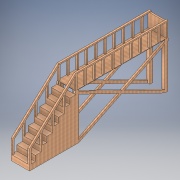
# Autodesk Inventor part: driver stand
Saved by Autodesk Inventor 2019 (Build 230136000, 136)
## iProperties
Created: 2020-04-29
Part Number: driver stand
Material: Wood (Birch)
Document SubType Name: Modeling
Designer: infinity
Density: 0.55 g/cm^3
Appearance: Birch - Natural Polished
Author: infinity
Autodesk Inventor part; units mm, degrees
ref_plane "YZ Plane" through (0, 0, 0) normal (1, 0, 0) x (0, 1, 0)
ref_plane "XZ Plane" through (0, 0, 0) normal (0, 1, 0) x (-1, 0, 0)
sketch "Sketch1" plane through (0, 0, 0) normal (0, 1, 0) x (-1, 0, 0)
  line L0 (0, 0) -> (1219.2, 0)
  line L1 (1219.2, 0) -> (1219.2, -6096)
  line L2 (1219.2, -6096) -> (0, -6096)
  line L3 (0, -6096) -> (0, 0)
  dimension "d0" = 6096
  dimension "d1" = 1219.2
  constraints: 8 end point, 2 parallel, 1 horizontal, 1 perpendicular
  measures "d0" distance of L0.end L1.end
  measures "d1" distance of L0.start L0.end
extrude "Extrusion1" add sketch "Sketch1" along normal blind 25.4
sketch "Sketch2" plane through (0, 0, 0) normal (0, -1, 0) x (1, 0, 0)
  line L0 (-1219.2, 0) -> (0, 0) projected
  line L1 (0, 0) -> (-203.2, 0)
  line L2 (-203.2, 0) -> (-203.2, -203.2)
  line L3 (-203.2, -203.2) -> (0, -203.2)
  line L4 (0, -203.2) -> (0, 0)
  line L5 (0, 0) -> (0, -6096) projected
  line L6 (0, -6096) -> (-203.2, -6096)
  line L7 (-203.2, -6096) -> (-203.2, -5892.8)
  line L8 (-203.2, -5892.8) -> (0, -5892.8)
  line L9 (0, -5892.8) -> (0, -6096)
  line L10 (0, -6096) -> (-1219.2, -6096) projected
  line L11 (-1219.2, -6096) -> (-994.7173, -6096)
  line L12 (-994.7173, -6096) -> (-994.7173, -5892.8)
  line L13 (-994.7173, -5892.8) -> (-1219.2, -5892.8)
  line L14 (-1219.2, -5892.8) -> (-1219.2, -6096)
  line L15 (-1219.2, 0) -> (-994.7173, 0)
  line L16 (-994.7173, 0) -> (-994.7173, -203.2)
  line L17 (-994.7173, -203.2) -> (-1219.2, -203.2)
  line L18 (-1219.2, -203.2) -> (-1219.2, 0)
  line L19 (-203.2, -203.2) -> (-994.7173, -203.2) construction
  line L20 (-994.7173, -203.2) -> (-994.7173, -5892.8) construction
  line L21 (-994.7173, -5892.8) -> (-203.2, -5892.8) construction
  line L22 (-203.2, -5892.8) -> (-203.2, -203.2) construction
  dimension "d4" = 203.2
  dimension "d5" = 203.2
  dimension "d6" = 203.2
  constraints: 40 end point, 10 parallel, 5 horizontal, 5 perpendicular, 5 point on line
  measures "d4" distance of L6.end L7.end
  measures "d5" distance of L5.end L6.end
  measures "d6" distance of L15.end L16.end
extrude "Extrusion2" add sketch "Sketch2" along normal blind 3048
sketch "Sketch3" plane through (0, 25.4, 0) normal (1, 0, 0) x (0, 0, -1)
  line L0 (5892.8, -3073.4) -> (-67.6758, -164.0495)
  line L1 (-67.6758, -164.0495) -> (0, -25.4)
  line L2 (0, -25.4) -> (5960.4758, -2934.7505)
  line L3 (5960.4758, -2934.7505) -> (5892.8, -3073.4)
  line L4 (5892.8, -3073.4) -> (0, -25.4) construction
  line L5 (-67.6758, -164.0495) -> (5960.4758, -2934.7505) construction
  line L6 (3048, 1078.3274) -> (3048, -3690.8651) construction
  line L7 (6096, 0) -> (6096, -3073.4) construction
  line L8 (0, -3073.4) -> (0, 0) construction
  line L9 (203.2, -3073.4) -> (6163.6758, -164.0495)
  line L10 (6163.6758, -164.0495) -> (6096, -25.4)
  line L11 (6096, -25.4) -> (135.5242, -2934.7505)
  line L12 (135.5242, -2934.7505) -> (203.2, -3073.4)
  line L13 (203.2, -3073.4) -> (6096, -25.4) construction
  line L14 (6163.6758, -164.0495) -> (135.5242, -2934.7505) construction
  line L15 (0, 0) -> (0, -3073.4) construction
  line L16 (6096, -3073.4) -> (6096, 0) construction
  point P0 (0, -25.4)
  point P1 (2946.4, -1549.4)
  point P2 (6096, -25.4)
  point P3 (3149.6, -1549.4)
  dimension "d9" = 6096
  dimension "d10" = 3048
  constraints: 30 end point, 11 symmetric about line, 4 coincident, 4 midpoint, 2 parallel, 1 perpendicular, 1 vertical
  measures "d9" distance between parallel lines of L7 L8
  measures "d10" distance between parallel lines of L6 L8
extrude "Extrusion3" add sketch "Sketch3" against normal blind 101.6
ref_plane "Work Plane1" through (-609.6, 25.4, 0) normal (1, 0, 0) x (0, 0, -1)
mirror "Mirror1" about plane through (-609.6, 25.4, 0) normal (1, 0, 0) of "Extrusion3"
sketch "Sketch4" plane through (-1219.2, 25.4, -6096) normal (-1, 0, 0) x (0, 0, 1)
  line L0 (6096, -197.0826) -> (6096, -3073.4) projected
  line L1 (6096, -3073.4) -> (9144, -3073.4)
  line L2 (9144, -3073.4) -> (9144, -2717.8)
  line L3 (9144, -2717.8) -> (8763, -2717.8)
  line L4 (8763, -2717.8) -> (8763, -2362.2)
  line L5 (8763, -2362.2) -> (8382, -2362.2)
  line L6 (8382, -2362.2) -> (8382, -2006.6)
  line L7 (8382, -2006.6) -> (8001, -2006.6)
  line L8 (8001, -2006.6) -> (8001, -1651)
  line L9 (8001, -1651) -> (7620, -1651)
  line L10 (7620, -1651) -> (7620, -1295.4)
  line L11 (7620, -1295.4) -> (7239, -1295.4)
  line L12 (7239, -1295.4) -> (7239, -939.8)
  line L13 (7239, -939.8) -> (6858, -939.8)
  line L14 (6858, -939.8) -> (6858, -584.2)
  line L15 (6858, -584.2) -> (6477, -584.2)
  line L16 (6477, -584.2) -> (6477, -228.6)
  line L17 (6477, -228.6) -> (6096, -228.6)
  point P0 (6096, -25.4)
  dimension "d13" = 381
  dimension "d14" = 381
  dimension "d15" = 381
  dimension "d16" = 381
  dimension "d17" = 381
  dimension "d18" = 381
  dimension "d19" = 381
  dimension "d20" = 381
  dimension "d21" = 355.6
  dimension "d22" = 355.6
  dimension "d23" = 355.6
  dimension "d24" = 355.6
  dimension "d25" = 355.6
  dimension "d26" = 355.6
  dimension "d27" = 355.6
  dimension "d57" = 355.6
  constraints: 34 end point, 16 perpendicular, 1 horizontal, 1 point on line
  measures "d13" distance of L16.end L17.end
  measures "d14" distance of L14.end L15.end
  measures "d15" distance of L12.end L13.end
  measures "d16" distance of L10.end L11.end
  measures "d17" distance of L8.end L9.end
  measures "d18" distance of L6.end L7.end
  measures "d19" distance of L4.end L5.end
  measures "d20" distance of L2.end L3.end
  measures "d21" distance of L15.end L16.end
  measures "d22" distance of L13.end L14.end
  measures "d23" distance of L11.end L12.end
  measures "d24" distance of L9.end L10.end
  measures "d25" distance of L7.end L8.end
  measures "d26" distance of L5.end L6.end
  measures "d27" distance of L3.end L4.end
  measures "d57" distance between parallel lines of L1 L3
extrude "Extrusion4" add sketch "Sketch4" against normal up to surface (1219.2 mm away)
sketch "Sketch5" plane through (0, 25.4, 0) normal (0, 1, 0) x (1, 0, 0)
  line L0 (-1219.2, 6096) -> (-1219.2, 0) projected
  line L1 (-1219.2, 0) -> (-1117.6, 0)
  line L2 (-1117.6, 0) -> (-1117.6, 101.6)
  line L3 (-1117.6, 101.6) -> (-1219.2, 101.6)
  line L4 (-1219.2, 101.6) -> (-1219.2, 0)
  line L5 (0, 0) -> (-101.6, 0)
  line L6 (-101.6, 0) -> (-101.6, 101.6)
  line L7 (-101.6, 101.6) -> (0, 101.6)
  line L8 (0, 101.6) -> (0, 0)
  line L9 (0, 5892.8) -> (0, 203.2) projected
  line L10 (-1219.2, 6096) -> (0, 6096)
  line L11 (0, 6096) -> (0, 5994.4)
  line L12 (0, 5994.4) -> (-1219.2, 5994.4)
  line L13 (-1219.2, 5994.4) -> (-1219.2, 6096)
  line L14 (-1117.6, 609.6) -> (-1117.6, 711.2)
  line L15 (-1219.2, 609.6) -> (-1117.6, 609.6)
  line L16 (-1117.6, 711.2) -> (-1219.2, 711.2)
  line L17 (-1219.2, 711.2) -> (-1219.2, 609.6)
  line L18 (0, 609.6) -> (-101.6, 609.6)
  line L19 (-101.6, 609.6) -> (-101.6, 711.2)
  line L20 (-101.6, 711.2) -> (0, 711.2)
  line L21 (0, 711.2) -> (0, 609.6)
  line L22 (-1117.6, 1219.2) -> (-1117.6, 1320.8)
  line L23 (-1219.2, 1219.2) -> (-1117.6, 1219.2)
  line L24 (-1117.6, 1320.8) -> (-1219.2, 1320.8)
  line L25 (-1219.2, 1320.8) -> (-1219.2, 1219.2)
  line L26 (0, 1219.2) -> (-101.6, 1219.2)
  line L27 (-101.6, 1219.2) -> (-101.6, 1320.8)
  line L28 (-101.6, 1320.8) -> (0, 1320.8)
  line L29 (0, 1320.8) -> (0, 1219.2)
  line L30 (-1117.6, 1828.8) -> (-1117.6, 1930.4)
  line L31 (-1219.2, 1828.8) -> (-1117.6, 1828.8)
  line L32 (-1117.6, 1930.4) -> (-1219.2, 1930.4)
  line L33 (-1219.2, 1930.4) -> (-1219.2, 1828.8)
  line L34 (0, 1828.8) -> (-101.6, 1828.8)
  line L35 (-101.6, 1828.8) -> (-101.6, 1930.4)
  line L36 (-101.6, 1930.4) -> (0, 1930.4)
  line L37 (0, 1930.4) -> (0, 1828.8)
  line L38 (-1117.6, 2438.4) -> (-1117.6, 2540)
  line L39 (-1219.2, 2438.4) -> (-1117.6, 2438.4)
  line L40 (-1117.6, 2540) -> (-1219.2, 2540)
  line L41 (-1219.2, 2540) -> (-1219.2, 2438.4)
  line L42 (0, 2438.4) -> (-101.6, 2438.4)
  line L43 (-101.6, 2438.4) -> (-101.6, 2540)
  line L44 (-101.6, 2540) -> (0, 2540)
  line L45 (0, 2540) -> (0, 2438.4)
  line L46 (-1117.6, 3048) -> (-1117.6, 3149.6)
  line L47 (-1219.2, 3048) -> (-1117.6, 3048)
  line L48 (-1117.6, 3149.6) -> (-1219.2, 3149.6)
  line L49 (-1219.2, 3149.6) -> (-1219.2, 3048)
  line L50 (0, 3048) -> (-101.6, 3048)
  line L51 (-101.6, 3048) -> (-101.6, 3149.6)
  line L52 (-101.6, 3149.6) -> (0, 3149.6)
  line L53 (0, 3149.6) -> (0, 3048)
  line L54 (-1117.6, 3657.6) -> (-1117.6, 3759.2)
  line L55 (-1219.2, 3657.6) -> (-1117.6, 3657.6)
  line L56 (-1117.6, 3759.2) -> (-1219.2, 3759.2)
  line L57 (-1219.2, 3759.2) -> (-1219.2, 3657.6)
  line L58 (0, 3657.6) -> (-101.6, 3657.6)
  line L59 (-101.6, 3657.6) -> (-101.6, 3759.2)
  line L60 (-101.6, 3759.2) -> (0, 3759.2)
  line L61 (0, 3759.2) -> (0, 3657.6)
  line L62 (-1117.6, 4267.2) -> (-1117.6, 4368.8)
  line L63 (-1219.2, 4267.2) -> (-1117.6, 4267.2)
  line L64 (-1117.6, 4368.8) -> (-1219.2, 4368.8)
  line L65 (-1219.2, 4368.8) -> (-1219.2, 4267.2)
  line L66 (0, 4267.2) -> (-101.6, 4267.2)
  line L67 (-101.6, 4267.2) -> (-101.6, 4368.8)
  line L68 (-101.6, 4368.8) -> (0, 4368.8)
  line L69 (0, 4368.8) -> (0, 4267.2)
  line L70 (-1117.6, 4876.8) -> (-1117.6, 4978.4)
  line L71 (-1219.2, 4876.8) -> (-1117.6, 4876.8)
  line L72 (-1117.6, 4978.4) -> (-1219.2, 4978.4)
  line L73 (-1219.2, 4978.4) -> (-1219.2, 4876.8)
  line L74 (0, 4876.8) -> (-101.6, 4876.8)
  line L75 (-101.6, 4876.8) -> (-101.6, 4978.4)
  line L76 (-101.6, 4978.4) -> (0, 4978.4)
  line L77 (0, 4978.4) -> (0, 4876.8)
  line L78 (-1117.6, 5486.4) -> (-1117.6, 5588)
  line L79 (-1219.2, 5486.4) -> (-1117.6, 5486.4)
  line L80 (-1117.6, 5588) -> (-1219.2, 5588)
  line L81 (-1219.2, 5588) -> (-1219.2, 5486.4)
  line L82 (0, 5486.4) -> (-101.6, 5486.4)
  line L83 (-101.6, 5486.4) -> (-101.6, 5588)
  line L84 (-101.6, 5588) -> (0, 5588)
  line L85 (0, 5588) -> (0, 5486.4)
  point P0 (0, 812.8)
  point P1 (0, 1422.4)
  point P2 (0, 2032)
  point P3 (0, 2641.6)
  point P4 (0, 3251.2)
  point P5 (0, 3860.8)
  point P6 (0, 4470.4)
  point P7 (0, 5080)
  point P8 (0, 5689.6)
  dimension "d30" = 101.6
  dimension "d31" = 101.6
  dimension "d32" = 101.6
  dimension "d33" = 101.6
  dimension "d34" = 101.6
  dimension "d39" = 609.6
  constraints: 168 end point, 6 parallel, 3 horizontal, 3 perpendicular, 1 point on line, 1 vertical, 153 other
  measures "d30" distance between parallel lines of L10 L12
  measures "d31" distance of L1.end L2.end
  measures "d32" distance of L6.end L7.end
  measures "d33" distance of L2.end L3.end
  measures "d34" distance of L7.end L5.start
  measures "d39" distance of L2.end L14.end
extrude "Extrusion5" add sketch "Sketch5" along normal blind 914.4
sketch "Sketch6" plane through (0, 939.8, 0) normal (0, 1, 0) x (1, 0, 0)
  line L0 (-1219.2, 6096) -> (-994.7173, 6096) projected
  line L1 (-1219.2, 0) -> (-1106.9586, 0)
  line L2 (-1106.9586, 0) -> (-1106.9586, 6096)
  line L3 (-1106.9586, 6096) -> (-1219.2, 6096)
  line L4 (-1219.2, 6096) -> (-1219.2, 0)
  line L5 (-203.2, 6096) -> (0, 6096) projected
  line L6 (-101.6, -67.6758) -> (-101.6, 0) projected
  line L7 (0, 6096) -> (-101.6, 6096)
  line L8 (-101.6, 6096) -> (-101.6, 0)
  line L9 (-101.6, 0) -> (0, 0)
  line L10 (0, 0) -> (0, 6096)
  point P0 (0, 0)
  constraints: 16 end point, 4 parallel, 2 horizontal, 2 perpendicular, 1 midpoint
extrude "Extrusion6" add sketch "Sketch6" along normal blind 76.2
sketch "Sketch7" plane through (0, -3048, 0) normal (0, -1, 0) x (1, 0, 0)
  line L0 (0, 3048) -> (0, 2667) projected
  line L1 (0, 3048) -> (-101.6, 3048)
  line L2 (-101.6, 3048) -> (-101.6, 2946.4)
  line L3 (-101.6, 2946.4) -> (0, 2946.4)
  line L4 (0, 2946.4) -> (0, 3048)
  line L5 (-1219.2, 2667) -> (-1219.2, 3048) projected
  line L6 (-1219.2, 3048) -> (-1117.6, 3048)
  line L7 (-1117.6, 3048) -> (-1117.6, 2946.4)
  line L8 (-1117.6, 2946.4) -> (-1219.2, 2946.4)
  line L9 (-1219.2, 2946.4) -> (-1219.2, 3048)
  line L10 (-1219.2, 2286) -> (-1117.6, 2286)
  line L11 (-1117.6, 2286) -> (-1117.6, 2184.4)
  line L12 (-1117.6, 2184.4) -> (-1219.2, 2184.4)
  line L13 (-1219.2, 2184.4) -> (-1219.2, 2286)
  line L14 (-1219.2, 2286) -> (0, 2286) projected
  line L15 (0, 2286) -> (-101.6, 2286)
  line L16 (-101.6, 2286) -> (-101.6, 2184.4)
  line L17 (-101.6, 2184.4) -> (0, 2184.4)
  line L18 (0, 2184.4) -> (0, 2286)
  line L19 (0, 1524) -> (-101.6, 1524)
  line L20 (-101.6, 1524) -> (-101.6, 1422.4)
  line L21 (-101.6, 1422.4) -> (0, 1422.4)
  line L22 (0, 1422.4) -> (0, 1524)
  line L23 (-1219.2, 1524) -> (-1219.2, 1905) projected
  line L24 (-1219.2, 1524) -> (-1117.6, 1524)
  line L25 (-1117.6, 1524) -> (-1117.6, 1422.4)
  line L26 (-1117.6, 1422.4) -> (-1219.2, 1422.4)
  line L27 (-1219.2, 1422.4) -> (-1219.2, 1524)
  line L28 (0, 762) -> (0, 381) projected
  line L29 (0, 762) -> (-101.6, 762)
  line L30 (-101.6, 762) -> (-101.6, 660.4)
  line L31 (-101.6, 660.4) -> (0, 660.4)
  line L32 (0, 660.4) -> (0, 762)
  line L33 (-1219.2, 762) -> (-1117.6, 762)
  line L34 (-1117.6, 762) -> (-1117.6, 660.4)
  line L35 (-1117.6, 660.4) -> (-1219.2, 660.4)
  line L36 (-1219.2, 660.4) -> (-1219.2, 762)
  point P0 (0, 0)
  dimension "d46" = 101.6
  dimension "d47" = 101.6
  dimension "d48" = 101.6
  dimension "d49" = 101.6
  dimension "d50" = 101.6
  dimension "d51" = 101.6
  dimension "d52" = 101.6
  dimension "d53" = 101.6
  dimension "d54" = 101.6
  constraints: 64 end point, 16 parallel, 8 horizontal, 8 perpendicular, 7 point on line
  measures "d46" distance of L0.start L1.end
  measures "d47" distance between parallel lines of L1 L3
  measures "d48" distance of L6.end L7.end
  measures "d49" distance of L7.end L8.end
  measures "d50" distance of L15.end L16.end
  measures "d51" distance of L19.end L20.end
  measures "d52" distance of L29.end L30.end
  measures "d53" distance between parallel lines of L36 L34
  measures "d54" distance between parallel lines of L27 L25
extrude "Extrusion7" add sketch "Sketch7" against normal blind 1270 contours L0 L3 L2 L1 | L5 L6 L7 L8
extrude "Extrusion8" add sketch "Sketch7" against normal blind 1981.2 contours L14 L18 L17 L16 | L10 L11 L12 L13
extrude "Extrusion9" add sketch "Sketch7" against normal blind 2692.4 contours L22 L21 L20 L19 | L24 L25 L26 L27
extrude "Extrusion10" add sketch "Sketch7" against normal blind 3403.6 contours L28 L31 L30 L29 | L33 L34 L35 L36
sketch "Sketch8" plane through (0, -3048, -6096) normal (1, 0, 0) x (0, 0, -1)
  line L0 (-9144, 1270) -> (-9042.4, 1270) projected
  line L1 (-6096, 3048) -> (-6096, 4064) projected
  line L2 (-9144, 1270) -> (-6096, 4064)
  line L3 (-6096, 4064) -> (-6011.6528, 3971.9849)
  line L4 (-6011.6528, 3971.9849) -> (-9059.6528, 1177.9849)
  line L5 (-9059.6528, 1177.9849) -> (-9144, 1270)
  constraints: 8 end point, 2 parallel, 1 perpendicular
extrude "Extrusion11" add sketch "Sketch8" against normal blind 101.6
mirror "Mirror2" about plane through (-609.6, 25.4, 0) normal (1, 0, 0) of "Extrusion11"
sketch "Sketch9" plane through (0, -3048, -6096) normal (1, 0, 0) x (0, 0, -1)
  line L0 (-9144, 1270) -> (-8382, 1968.5) projected
  line L1 (-9144, 1270) -> (-6096, 4064)
  line L2 (-6096, 4064) -> (-6333.3878, 4505.2973)
  line L3 (-6333.3878, 4505.2973) -> (-9428.221, 1744.5652)
  line L4 (-9144, 355.6) -> (-9144, 1270) projected
  line L5 (-9428.221, 1744.5652) -> (-9144, 1270)
  point P0 (-6096, 3048)
  constraints: 8 end point, 1 collinear
extrude "Extrusion12" cut sketch "Sketch9" along normal through all both and the other way through all
equation "\"d5\" = d4"
equation "\"d6\" = d5"
equation "\"d10\" = 0.5 * d9"
equation "\"d14\" = d13"
equation "\"d15\" = d14"
equation "\"d16\" = d15"
equation "\"d17\" = d16"
equation "\"d18\" = d17"
equation "\"d19\" = d18"
equation "\"d20\" = d19"
equation "\"d22\" = d21"
equation "\"d23\" = d21"
equation "\"d24\" = d21"
equation "\"d25\" = d24"
equation "\"d26\" = d25"
equation "\"d27\" = d26"
equation "\"d57\" = d27"
equation "\"d47\" = d46"
equation "\"d48\" = d47"
equation "\"d49\" = d47"
equation "\"d50\" = d47"
equation "\"d51\" = d50"
equation "\"d52\" = d50"
equation "\"d53\" = d51"
equation "\"d54\" = d53"
body "Solid1"
